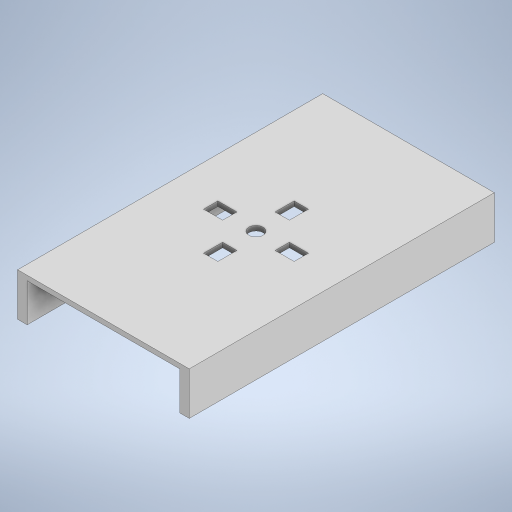
# Autodesk Inventor part: Guide for 2in box tube
Saved by Autodesk Inventor 2023 (Build 270158000, 158)
## iProperties
Created: 2023-01-21
Part Number: Guide for 2in box tube
Material: Generic
Document SubType Name: Modeling
Designer: Gabriel - T3 CAD
Density: 1 g/cm^3
Appearance: Default
Author: Gabriel - T3 CAD
Autodesk Inventor part; units mm, degrees
ref_plane "YZ Plane" through (0, 0, 0) normal (1, 0, 0) x (0, 1, 0)
ref_plane "XZ Plane" through (0, 0, 0) normal (0, 1, 0) x (-1, 0, 0)
ref_plane "XY Plane" through (0, 0, 0) normal (0, 0, 1) x (1, 0, 0)
sketch "Sketch1" plane through (0, 0, 0) normal (0, 1, 0) x (-1, 0, 0)
  line L0 (0, 0) -> (50.8, 0)
  line L1 (50.8, 0) -> (50.8, 101.6)
  line L2 (50.8, 101.6) -> (0, 101.6)
  line L3 (0, 101.6) -> (0, 0)
  line L4 (50.8, 101.6) -> (53.975, 101.6)
  line L5 (53.975, 101.6) -> (53.975, 0)
  line L6 (53.975, 0) -> (50.8, 0)
  line L7 (50.8, 0) -> (50.8, 101.6)
  line L8 (0, 101.6) -> (-3.175, 101.6)
  line L9 (-3.175, 101.6) -> (-3.175, 0)
  line L10 (-3.175, 0) -> (0, 0)
  line L11 (0, 0) -> (0, 101.6)
  circle A0 centre (25.4, 50.8) radius 2.3813
  line L12 (50.8, 53.1813) -> (0, 53.1813)
  line L13 (0, 53.1813) -> (0, 48.4188)
  line L14 (0, 48.4188) -> (50.8, 48.4188)
  line L15 (50.8, 48.4188) -> (50.8, 53.1813)
  line L16 (27.7813, 101.6) -> (23.0188, 101.6)
  line L17 (23.0188, 101.6) -> (23.0188, 0)
  line L18 (23.0188, 0) -> (27.7813, 0)
  line L19 (27.7813, 0) -> (27.7813, 101.6)
  line L20 (27.7812, 65.8812) -> (23.0187, 65.8812)
  line L21 (23.0187, 65.8812) -> (23.0187, 59.5312)
  line L22 (23.0187, 59.5312) -> (27.7812, 59.5312)
  line L23 (27.7812, 59.5312) -> (27.7812, 65.8812)
  line L24 (40.4812, 53.1813) -> (34.1313, 53.1813)
  line L25 (34.1313, 53.1813) -> (34.1313, 48.4188)
  line L26 (34.1313, 48.4188) -> (40.4812, 48.4188)
  line L27 (40.4812, 48.4188) -> (40.4812, 53.1813)
  line L28 (27.7812, 42.0688) -> (23.0187, 42.0688)
  line L29 (23.0187, 42.0688) -> (23.0188, 35.7188)
  line L30 (23.0188, 35.7188) -> (27.7812, 35.7188)
  line L31 (27.7812, 35.7188) -> (27.7812, 42.0688)
  line L32 (16.6687, 53.1813) -> (10.3187, 53.1813)
  line L33 (10.3187, 53.1813) -> (10.3188, 48.4188)
  line L34 (10.3188, 48.4188) -> (16.6688, 48.4188)
  line L35 (16.6688, 48.4188) -> (16.6687, 53.1813)
  point P0 (0, 50.8)
  point P1 (25.4, 53.1813)
  point P2 (25.4, 35.7188)
  point P3 (25.4, 42.0688)
  dimension "d0" = 50.8
  dimension "d1" = 101.6
  dimension "d2" = 3.175
  dimension "d3" = 101.6
  dimension "d4" = 3.175
  dimension "d5" = 101.6
  dimension "d6" = 4.7625
  dimension "d7" = 25.4
  dimension "d8" = 50.8
  dimension "d9" = 4.7625
  dimension "d10" = 4.7625
  dimension "d11" = 2.3813
  dimension "d12" = 2.3813
  dimension "d13" = 6.35
  dimension "d14" = 6.35
  dimension "d15" = 6.35
  dimension "d16" = 6.35
  dimension "d17" = 6.35
  dimension "d18" = 6.35
  dimension "d19" = 6.35
  dimension "d20" = 6.35
  constraints: 72 end point, 18 parallel, 12 point on line, 9 horizontal, 9 perpendicular, 4 midpoint, 1 centre point
  measures "d0" distance of L2.end L1.end
  measures "d1" distance of L1.end L0.end
  measures "d2" distance of L5.end L6.end
  measures "d3" distance of L4.end L5.end
  measures "d4" distance of L10.end L9.end
  measures "d5" distance of L9.end L8.end
  measures "d6" diameter of A0
  measures "d7" distance of point (0, 50.8) A0.centre
  measures "d8" distance from line of L2 A0.centre
  measures "d9" distance between parallel lines of L17 L19
  measures "d10" distance between parallel lines of L12 L14
  measures "d11" distance of A0.centre point (25.4, 53.181)
  measures "d12" distance from line of A0.centre L19
  measures "d13" distance of L33.end L34.end
  measures "d14" distance of point (25.4, 35.719) point (25.4, 42.069)
  measures "d15" distance of L24.start L24.end
  measures "d16" distance between parallel lines of L20 L22
  measures "d17" distance between parallel lines of L12 L22
  measures "d18" distance between parallel lines of L19 L25
  measures "d19" distance from line of L14 point (25.4, 42.069)
  measures "d20" distance between parallel lines of L17 L35
extrude "Extrusion1" add sketch "Sketch1" along normal blind 1.5875 contours L3 L14 L17 L0 | L17 L30 L19 L0 | L3 L12 L33 L14 | L19 L14 L1 L0 | L3 L2 L17 L12 | L17 L14 L19 L28 | L35 L12 L17 L14 | L14 L27 L12 L1 | L17 A0 L14 | L2 L19 L20 L17 | L12 L19 L2 L1 | L19 L12 L25 L14 | L14 A0 L19 | L17 L12 A0 | L17 L22 L19 L12 | A0 L12 L19
extrude "Extrusion2" add sketch "Sketch1" along normal blind 1.5875 and the other way blind 12.7 contours L10 L9 L8 L3 | L1 L4 L5 L6
equation "\"d11\" = 0.5 * d6"
equation "\"d12\" = 0.5 * d6"
equation "\"d15\" = d14"
equation "\"d16\" = d15"
body "Solid1"
